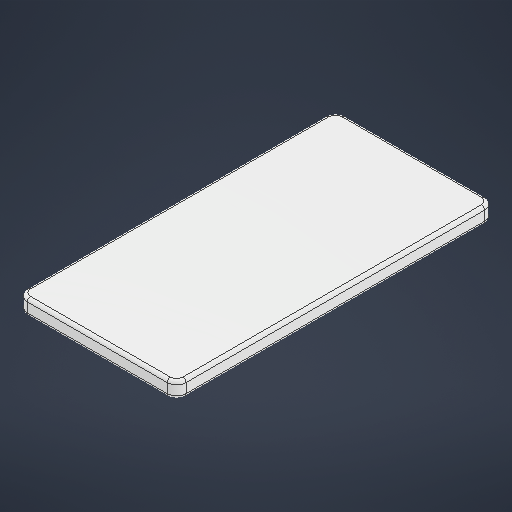
# Autodesk Inventor part: battery-5050100_4000
Saved by Autodesk Inventor 2025.2 (Build 292293000, 293)
## iProperties
Created: 2025-12-22
Part Number: battery-5050100_4000
Material: PC/ABS Plastic
Document SubType Name: Modeling
Designer: sam
Density: 1.1 g/cm^3
Appearance: Smooth - White
Author: sam
Autodesk Inventor part; units mm, degrees
ref_plane "YZ Plane" through (0, 0, 0) normal (1, 0, 0) x (0, 1, 0)
ref_plane "XZ Plane" through (0, 0, 0) normal (0, 1, 0) x (-1, 0, 0)
ref_plane "XY Plane" through (0, 0, 0) normal (0, 0, 1) x (1, 0, 0)
sketch "Sketch1" plane through (0, 0, 0) normal (0, 1, 0) x (-1, 0, 0)
  line L0 (-25, -50) -> (25, -50)
  line L1 (25, -50) -> (25, 50)
  line L2 (25, 50) -> (-25, 50)
  line L3 (-25, 50) -> (-25, -50)
  line L4 (-25, -50) -> (25, 50) construction
  line L5 (25, -50) -> (-25, 50) construction
  point P0 (0, 0)
  dimension "d0" = 50
  dimension "d1" = 100
  constraints: 12 end point, 2 midpoint, 2 parallel, 1 horizontal, 1 perpendicular
  measures "d0" distance of L2.end L1.end
  measures "d1" distance of L1.end L0.end
extrude "Extrusion1" add sketch "Sketch1" along normal blind 5
fillet "Fillet1" radius 1 8 edges at (0, 5, 50) (0, 0, 50) (0, 5, -50) (0, 0, -50) (25, 5, 0) (25, 0, 0) (-25, 5, 0) (-25, 0, 0)
fillet "Fillet2" radius 3 12 edges at (24.7071, 4.7071, -49.7071) (24.7071, 0.2929, -49.7071) (25, 2.5, -50) (-24.7071, 4.7071, -49.7071) (-24.7071, 0.2929, -49.7071) (-25, 2.5, -50) (-24.7071, 4.7071, 49.7071) (-24.7071, 0.2929, 49.7071) (-25, 2.5, 50) (24.7071, 4.7071, 49.7071) (24.7071, 0.2929, 49.7071) (25, 2.5, 50)
body "Solid1"
